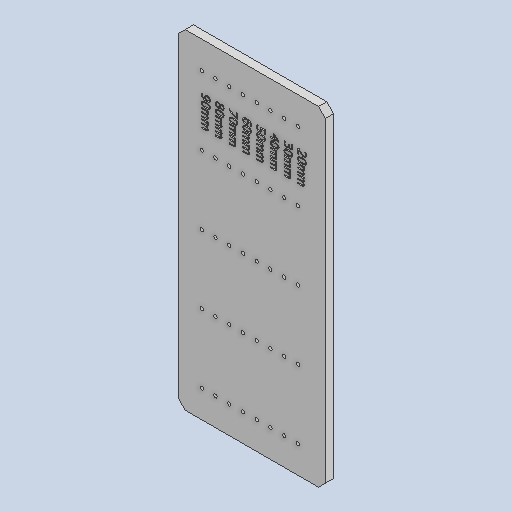
# Autodesk Inventor part: A-01
Saved by Autodesk Inventor 2022 (Build 260153000, 153)
## iProperties
Created: 2021-10-10
Part Number: A-01
Material: Generic
Document SubType Name: Modeling
Designer: kfcs7
Density: 1 g/cm^3
Appearance: Default
Author: kfcs7
Autodesk Inventor part; units mm, degrees
(part 1 of 2)
ref_plane "YZ Plane" through (0, 0, 0) normal (1, 0, 0) x (0, 1, 0)
ref_plane "XZ Plane" through (0, 0, 0) normal (0, 1, 0) x (-1, 0, 0)
ref_plane "XY Plane" through (0, 0, 0) normal (0, 0, 1) x (1, 0, 0)
sketch "Sketch1" plane through (0, 0, 0) normal (0, 0, 1) x (1, 0, 0)
  line L0 (14.5, -5) -> (14.5, -245) construction
  line L1 (14.5, -5) -> (0, -5) construction
  line L2 (0, -5) -> (0, -245) construction
  line L3 (0, -245) -> (14.5, -245) construction
  circle A0 centre (7, -25) radius 3.75 construction
  circle A1 centre (7, -75) radius 3.75 construction
  circle A2 centre (7, -125) radius 3.75 construction
  circle A3 centre (7, -175) radius 3.75 construction
  circle A4 centre (7, -225) radius 3.75 construction
  line L4 (27, -5) -> (-80, -5)
  line L5 (-80, -5) -> (-80, -245)
  line L6 (-80, -245) -> (27, -245)
  line L7 (27, -245) -> (27, -5)
  point P0 (0, 0)
  dimension "d6" = 20
  dimension "d9" = 80
  constraints: 8 end point, 2 collinear, 2 parallel, 1 horizontal, 1 perpendicular
  measures "d6" distance from line of L7 A0.centre
  measures "d9" distance between parallel lines of L2 L5
extrude "Extrusion1" add sketch "Sketch1" along normal blind 6
sketch "Sketch3" plane through (0, 0, 6) normal (0, 0, 1) x (1, 0, 0)
  line L0 (14.5, -5) -> (14.5, -245) construction
  line L1 (14.5, -5) -> (0, -5) construction
  line L2 (0, -5) -> (0, -245) construction
  line L3 (0, -245) -> (14.5, -245) construction
  circle A0 centre (7, -25) radius 3.75 construction
  circle A1 centre (7, -75) radius 3.75 construction
  circle A2 centre (7, -125) radius 3.75 construction
  circle A3 centre (7, -175) radius 3.75 construction
  circle A4 centre (7, -225) radius 3.75 construction
  circle A5 centre (7, -25) radius 1.25
  circle A6 centre (7, -75) radius 1.25
  circle A7 centre (7, -125) radius 1.25
  circle A8 centre (7, -175) radius 1.25
  circle A9 centre (7, -225) radius 1.25
  point P0 (0, 0)
  dimension "d10" = 2.5
  dimension "d11" = 2.5
  dimension "d12" = 2.5
  dimension "d13" = 2.5
  dimension "d14" = 2.5
  constraints: 5 centre point, 5 coincident
  measures "d10" diameter of A5
  measures "d11" diameter of A6
  measures "d12" diameter of A7
  measures "d13" diameter of A8
  measures "d14" diameter of A9
extrude "Extrusion2" cut sketch "Sketch3" against normal through all
chamfer "Chamfer1" distance 5 angle 45 4 edges at (27, -5, 3) (-80, -5, 3) (-80, -245, 3) (27, -245, 3)
pattern_linear "Rectangular Pattern1" count 8 spacing 10 along (-1, 0, 0) of "Extrusion2"
sketch "Sketch4" plane through (0, 0, 6) normal (0, 0, 1) x (1, 0, 0)
  circle A0 centre (7, -75) radius 1.25 construction
  circle A1 centre (7, -175) radius 1.25 construction
  circle A2 centre (7, -125) radius 1.25 construction
  circle A3 centre (7, -25) radius 1.25 construction
  circle A4 centre (7, -225) radius 1.25 construction
  line L0 (-80, -10) -> (-80, -240) construction
  line L1 (-75, -245) -> (22, -245) construction
  line L2 (27, -240) -> (27, -10) construction
  line L3 (22, -5) -> (-75, -5) construction
  circle A5 centre (7, -25) radius 1.25 construction
  circle A6 centre (7, -75) radius 1.25 construction
  line L4 (7, -25) -> (7, -75) construction
  line L5 (27, -240) -> (22, -245) construction
  line L6 (22, -5) -> (27, -10) construction
  line L7 (-80, -10) -> (-75, -5) construction
  line L8 (-75, -245) -> (-80, -240) construction
  circle A7 centre (-63, -75) radius 1.25 construction
  circle A8 centre (-63, -225) radius 1.25 construction
  circle A9 centre (-63, -25) radius 1.25 construction
  circle A10 centre (-63, -125) radius 1.25 construction
  circle A11 centre (-63, -175) radius 1.25 construction
  circle A12 centre (-53, -75) radius 1.25 construction
  circle A13 centre (-53, -225) radius 1.25 construction
  circle A14 centre (-53, -25) radius 1.25 construction
  circle A15 centre (-53, -125) radius 1.25 construction
  circle A16 centre (-53, -175) radius 1.25 construction
  circle A17 centre (-43, -75) radius 1.25 construction
  circle A18 centre (-43, -225) radius 1.25 construction
  circle A19 centre (-43, -25) radius 1.25 construction
  circle A20 centre (-43, -125) radius 1.25 construction
  circle A21 centre (-43, -175) radius 1.25 construction
  circle A22 centre (-33, -75) radius 1.25 construction
  circle A23 centre (-33, -225) radius 1.25 construction
  circle A24 centre (-33, -25) radius 1.25 construction
  circle A25 centre (-33, -125) radius 1.25 construction
  circle A26 centre (-33, -175) radius 1.25 construction
  circle A27 centre (-23, -75) radius 1.25 construction
  circle A28 centre (-23, -225) radius 1.25 construction
  circle A29 centre (-23, -25) radius 1.25 construction
  circle A30 centre (-23, -125) radius 1.25 construction
  circle A31 centre (-23, -175) radius 1.25 construction
  circle A32 centre (-13, -75) radius 1.25 construction
  circle A33 centre (-13, -225) radius 1.25 construction
  circle A34 centre (-13, -25) radius 1.25 construction
  circle A35 centre (-13, -125) radius 1.25 construction
  circle A36 centre (-13, -175) radius 1.25 construction
  circle A37 centre (-3, -75) radius 1.25 construction
  circle A38 centre (-3, -225) radius 1.25 construction
  circle A39 centre (-3, -25) radius 1.25 construction
  circle A40 centre (-3, -125) radius 1.25 construction
  circle A41 centre (-3, -175) radius 1.25 construction
  line L9 (27, -240) -> (22, -245) construction
  line L10 (27, -240) -> (27, -10) construction
  line L11 (22, -5) -> (27, -10) construction
  line L12 (22, -5) -> (-75, -5) construction
  line L13 (-80, -10) -> (-75, -5) construction
  line L14 (-80, -10) -> (-80, -240) construction
  line L15 (-75, -245) -> (-80, -240) construction
  line L16 (-75, -245) -> (22, -245) construction
  circle A42 centre (7, -75) radius 1.25 construction
  circle A43 centre (7, -175) radius 1.25 construction
  circle A44 centre (7, -125) radius 1.25 construction
  circle A45 centre (7, -25) radius 1.25 construction
  circle A46 centre (7, -225) radius 1.25 construction
  circle A47 centre (-3, -25) radius 1.25 construction
  line L17 (-3, -25) -> (-3, -75) construction
  circle A48 centre (-13, -75) radius 1.25 construction
  line L18 (-13, -25) -> (-13, -75) construction
  circle A49 centre (-23, -75) radius 1.25 construction
  circle A50 centre (-23, -25) radius 1.25 construction
  line L19 (-23, -75) -> (-23, -25) construction
  circle A51 centre (-33, -25) radius 1.25 construction
  circle A52 centre (-33, -75) radius 1.25 construction
  line L20 (-33, -25) -> (-33, -75) construction
  circle A53 centre (-43, -75) radius 1.25 construction
  circle A54 centre (-43, -25) radius 1.25 construction
  line L21 (-43, -75) -> (-43, -25) construction
  circle A55 centre (-53, -25) radius 1.25 construction
  circle A56 centre (-53, -75) radius 1.25 construction
  line L22 (-53, -25) -> (-53, -75) construction
  circle A57 centre (-63, -25) radius 1.25 construction
  circle A58 centre (-63, -75) radius 1.25 construction
  line L23 (-63, -25) -> (-63, -75) construction
  line L24 (7, -42.5851) -> (7, -38.8233)
  line L25 (7, -38.8233) -> (7.8651, -38.8233)
  spline S0 degree 2 poles (7.8651, -38.8233) (8.2457, -39.2286) (8.9526, -39.9503) (9.3332, -40.2964) knots 0 0 0 1 2 2 2
  spline S1 degree 2 poles (9.3332, -40.2964) (10.0994, -40.9934) (11.0189, -41.5025) (11.5083, -41.5025) knots 0 0 0 1 2 2 2
  spline S2 degree 2 poles (11.5083, -41.5025) (11.7653, -41.5025) (12.1509, -41.3443) (12.2745, -41.201) knots 0 0 0 1 2 2 2
  spline S3 degree 2 poles (12.2745, -41.201) (12.3981, -41.0576) (12.5216, -40.6819) (12.5216, -40.4545) knots 0 0 0 1 2 2 2
  spline S4 degree 2 poles (12.5216, -40.4545) (12.5216, -40.237) (12.4129, -39.7921) (12.3288, -39.5895) knots 0 0 0 1 2 2 2
  spline S5 degree 2 poles (12.3288, -39.5895) (12.2596, -39.4165) (12.0619, -39.0951) (11.9927, -38.9963) knots 0 0 0 1 2 2 2
  line L26 (11.9927, -38.9963) -> (11.9927, -38.9518)
  line L27 (11.9927, -38.9518) -> (12.8627, -38.9518)
  spline S6 degree 2 poles (12.8627, -38.9518) (12.9863, -39.2039) (13.2285, -40.1085) (13.2285, -40.5139) knots 0 0 0 1 2 2 2
  spline S7 degree 2 poles (13.2285, -40.5139) (13.2285, -41.369) (12.3239, -42.333) (11.5528, -42.333) knots 0 0 0 1 2 2 2
  spline S8 degree 2 poles (11.5528, -42.333) (11.1919, -42.333) (10.5888, -42.1649) (10.3318, -42.0166) knots 0 0 0 1 2 2 2
  spline S9 degree 2 poles (10.3318, -42.0166) (10.0648, -41.8683) (9.5408, -41.4382) (9.2887, -41.201) knots 0 0 0 1 2 2 2
  spline S10 degree 2 poles (9.2887, -41.201) (8.8686, -40.8154) (7.9689, -39.8712) (7.7069, -39.5895) knots 0 0 0 1 2 2 2
  line L28 (7.7069, -39.5895) -> (7.7069, -42.5851)
  line L29 (7.7069, -42.5851) -> (7, -42.5851)
  spline S11 degree 2 poles (10.05, -47.1972) (8.4088, -47.1972) (6.8715, -46.2431) (6.8715, -45.2495) knots 0 0 0 1 2 2 2
  spline S12 degree 2 poles (6.8715, -45.2495) (6.8715, -44.2411) (8.4385, -43.2969) (10.0451, -43.2969) knots 0 0 0 1 2 2 2
  spline S13 degree 2 poles (10.0451, -43.2969) (11.6961, -43.2969) (13.2236, -44.251) (13.2236, -45.2495) knots 0 0 0 1 2 2 2
  spline S14 degree 2 poles (13.2236, -45.2495) (13.2236, -46.253) (11.6417, -47.1972) (10.05, -47.1972) knots 0 0 0 1 2 2 2
  spline S15 degree 2 poles (8.1913, -46.1492) (8.4929, -46.2678) (9.4222, -46.3667) (10.05, -46.3667) knots 0 0 0 1 2 2 2
  spline S16 degree 2 poles (10.05, -46.3667) (10.6778, -46.3667) (11.6022, -46.2678) (11.9136, -46.1442) knots 0 0 0 1 2 2 2
  spline S17 degree 2 poles (11.9136, -46.1442) (12.225, -46.0207) (12.5464, -45.5906) (12.5464, -45.2495) knots 0 0 0 1 2 2 2
  spline S18 degree 2 poles (12.5464, -45.2495) (12.5464, -44.9084) (12.225, -44.4685) (11.9037, -44.34) knots 0 0 0 1 2 2 2
  spline S19 degree 2 poles (11.9037, -44.34) (11.5923, -44.2164) (10.6432, -44.1274) (10.0451, -44.1274) knots 0 0 0 1 2 2 2
  spline S20 degree 2 poles (10.0451, -44.1274) (9.4024, -44.1274) (8.5423, -44.2065) (8.2062, -44.335) knots 0 0 0 1 2 2 2
  spline S21 degree 2 poles (8.2062, -44.335) (7.8898, -44.4536) (7.5487, -44.8936) (7.5487, -45.2495) knots 0 0 0 1 2 2 2
  spline S22 degree 2 poles (7.5487, -45.2495) (7.5487, -45.5857) (7.87, -46.0256) (8.1913, -46.1492) knots 0 0 0 1 2 2 2
  line L30 (7, -53.2823) -> (9.6496, -53.2823)
  spline S23 degree 2 poles (9.6496, -53.2823) (9.966, -53.2823) (10.5048, -53.2329) (10.6531, -53.1538) knots 0 0 0 1 2 2 2
  spline S24 degree 2 poles (10.6531, -53.1538) (10.8162, -53.0747) (10.9744, -52.7732) (10.9744, -52.5112) knots 0 0 0 1 2 2 2
  spline S25 degree 2 poles (10.9744, -52.5112) (10.9744, -52.2739) (10.6827, -51.7301) (10.4059, -51.4434) knots 0 0 0 1 2 2 2
  spline S26 degree 2 poles (10.4059, -51.4434) (10.3367, -51.4484) (10.1439, -51.4583) (10.0154, -51.4583) knots 0 0 0 1 2 2 2
  line L31 (10.0154, -51.4583) -> (7, -51.4583)
  line L32 (7, -51.4583) -> (7, -50.6871)
  line L33 (7, -50.6871) -> (9.6496, -50.6871)
  spline S27 degree 2 poles (9.6496, -50.6871) (9.966, -50.6871) (10.5048, -50.6377) (10.6531, -50.5586) knots 0 0 0 1 2 2 2
  spline S28 degree 2 poles (10.6531, -50.5586) (10.8162, -50.4795) (10.9744, -50.178) (10.9744, -49.916) knots 0 0 0 1 2 2 2
  spline S29 degree 2 poles (10.9744, -49.916) (10.9744, -49.6688) (10.663, -49.1201) (10.4207, -48.863) knots 0 0 0 1 2 2 2
  line L34 (10.4207, -48.863) -> (7, -48.863)
  line L35 (7, -48.863) -> (7, -48.0919)
  line L36 (7, -48.0919) -> (11.5775, -48.0919)
  line L37 (11.5775, -48.0919) -> (11.5775, -48.863)
  line L38 (11.5775, -48.863) -> (11.0733, -48.863)
  spline S30 degree 2 poles (11.0733, -48.863) (11.3748, -49.1646) (11.706, -49.7578) (11.706, -50.1137) knots 0 0 0 1 2 2 2
  spline S31 degree 2 poles (11.706, -50.1137) (11.706, -50.519) (11.3353, -51.1468) (10.9151, -51.31) knots 0 0 0 1 2 2 2
  spline S32 degree 2 poles (10.9151, -51.31) (11.3056, -51.6609) (11.706, -52.3233) (11.706, -52.7089) knots 0 0 0 1 2 2 2
  spline S33 degree 2 poles (11.706, -52.7089) (11.706, -53.0055) (11.5231, -53.49) (11.3155, -53.6679) knots 0 0 0 1 2 2 2
  spline S34 degree 2 poles (11.3155, -53.6679) (11.1079, -53.8508) (10.485, -54.0535) (10.0154, -54.0535) knots 0 0 0 1 2 2 2
  line L39 (10.0154, -54.0535) -> (7, -54.0535)
  line L40 (7, -54.0535) -> (7, -53.2823)
  line L41 (7, -60.3265) -> (9.6496, -60.3265)
  spline S35 degree 2 poles (9.6496, -60.3265) (9.966, -60.3265) (10.5048, -60.2771) (10.6531, -60.198) knots 0 0 0 1 2 2 2
  spline S36 degree 2 poles (10.6531, -60.198) (10.8162, -60.1189) (10.9744, -59.8173) (10.9744, -59.5553) knots 0 0 0 1 2 2 2
  spline S37 degree 2 poles (10.9744, -59.5553) (10.9744, -59.3181) (10.6827, -58.7743) (10.4059, -58.4876) knots 0 0 0 1 2 2 2
  spline S38 degree 2 poles (10.4059, -58.4876) (10.3367, -58.4925) (10.1439, -58.5024) (10.0154, -58.5024) knots 0 0 0 1 2 2 2
  line L42 (10.0154, -58.5024) -> (7, -58.5024)
  line L43 (7, -58.5024) -> (7, -57.7313)
  line L44 (7, -57.7313) -> (9.6496, -57.7313)
  spline S39 degree 2 poles (9.6496, -57.7313) (9.966, -57.7313) (10.5048, -57.6818) (10.6531, -57.6028) knots 0 0 0 1 2 2 2
  spline S40 degree 2 poles (10.6531, -57.6028) (10.8162, -57.5237) (10.9744, -57.2221) (10.9744, -56.9601) knots 0 0 0 1 2 2 2
  spline S41 degree 2 poles (10.9744, -56.9601) (10.9744, -56.713) (10.663, -56.1643) (10.4207, -55.9072) knots 0 0 0 1 2 2 2
  line L45 (10.4207, -55.9072) -> (7, -55.9072)
  line L46 (7, -55.9072) -> (7, -55.1361)
  line L47 (7, -55.1361) -> (11.5775, -55.1361)
  line L48 (11.5775, -55.1361) -> (11.5775, -55.9072)
  line L49 (11.5775, -55.9072) -> (11.0733, -55.9072)
  spline S42 degree 2 poles (11.0733, -55.9072) (11.3748, -56.2088) (11.706, -56.8019) (11.706, -57.1579) knots 0 0 0 1 2 2 2
  spline S43 degree 2 poles (11.706, -57.1579) (11.706, -57.5632) (11.3353, -58.191) (10.9151, -58.3541) knots 0 0 0 1 2 2 2
  spline S44 degree 2 poles (10.9151, -58.3541) (11.3056, -58.7051) (11.706, -59.3675) (11.706, -59.7531) knots 0 0 0 1 2 2 2
  spline S45 degree 2 poles (11.706, -59.7531) (11.706, -60.0497) (11.5231, -60.5341) (11.3155, -60.7121) knots 0 0 0 1 2 2 2
  spline S46 degree 2 poles (11.3155, -60.7121) (11.1079, -60.895) (10.485, -61.0976) (10.0154, -61.0976) knots 0 0 0 1 2 2 2
  line L50 (10.0154, -61.0976) -> (7, -61.0976)
  line L51 (7, -61.0976) -> (7, -60.3265)
  spline S47 degree 2 poles (2.5216, -40.4694) (2.5216, -40.2469) (2.4129, -39.807) (2.3288, -39.5944) knots 0 0 0 1 2 2 2
  spline S48 degree 2 poles (2.3288, -39.5944) (2.2448, -39.3967) (2.0669, -39.105) (1.9878, -38.9913) knots 0 0 0 1 2 2 2
  line L52 (1.9878, -38.9913) -> (1.9878, -38.9419)
  line L53 (1.9878, -38.9419) -> (2.8528, -38.9419)
  spline S49 degree 2 poles (2.8528, -38.9419) (2.9962, -39.2088) (3.2285, -40.1233) (3.2285, -40.5336) knots 0 0 0 1 2 2 2
  spline S50 degree 2 poles (3.2285, -40.5336) (3.2285, -40.9489) (3.0605, -41.5668) (2.8825, -41.8189) knots 0 0 0 1 2 2 2
  spline S51 degree 2 poles (2.8825, -41.8189) (2.6897, -42.0858) (2.1311, -42.3626) (1.7554, -42.3626) knots 0 0 0 1 2 2 2
  spline S52 degree 2 poles (1.7554, -42.3626) (1.2512, -42.3626) (0.49, -41.7002) (0.3911, -41.2356) knots 0 0 0 1 2 2 2
  line L54 (0.3911, -41.2356) -> (0.3318, -41.2356)
  spline S53 degree 2 poles (0.3318, -41.2356) (0.2922, -41.4284) (0.1143, -41.8683) (-0.0637, -42.0562) knots 0 0 0 1 2 2 2
  spline S54 degree 2 poles (-0.0637, -42.0562) (-0.2367, -42.244) (-0.7904, -42.4813) (-1.1908, -42.4813) knots 0 0 0 1 2 2 2
  spline S55 degree 2 poles (-1.1908, -42.4813) (-1.6011, -42.4813) (-2.2981, -42.1995) (-2.565, -41.9425) knots 0 0 0 1 2 2 2
  spline S56 degree 2 poles (-2.565, -41.9425) (-2.8418, -41.6755) (-3.1285, -40.9192) (-3.1285, -40.4397) knots 0 0 0 1 2 2 2
  spline S57 degree 2 poles (-3.1285, -40.4397) (-3.1285, -39.98) (-2.9061, -39.0803) (-2.7528, -38.7738) knots 0 0 0 1 2 2 2
  line L55 (-2.7528, -38.7738) -> (-1.8878, -38.7738)
  line L56 (-1.8878, -38.7738) -> (-1.8878, -38.8331)
  spline S58 degree 2 poles (-1.8878, -38.8331) (-2.0756, -39.0902) (-2.4216, -39.9602) (-2.4216, -40.3903) knots 0 0 0 1 2 2 2
  spline S59 degree 2 poles (-2.4216, -40.3903) (-2.4216, -40.6424) (-2.2635, -41.1466) (-2.0806, -41.3147) knots 0 0 0 1 2 2 2
  spline S60 degree 2 poles (-2.0806, -41.3147) (-1.8976, -41.4778) (-1.4626, -41.6508) (-1.1314, -41.6508) knots 0 0 0 1 2 2 2
  spline S61 degree 2 poles (-1.1314, -41.6508) (-0.8002, -41.6508) (-0.3702, -41.458) (-0.2466, -41.285) knots 0 0 0 1 2 2 2
  spline S62 degree 2 poles (-0.2466, -41.285) (-0.123, -41.112) (-0.0291, -40.6424) (-0.0291, -40.3656) knots 0 0 0 1 2 2 2
  line L57 (-0.0291, -40.3656) -> (-0.0291, -40.0195)
  line L58 (-0.0291, -40.0195) -> (0.6481, -40.0195)
  line L59 (0.6481, -40.0195) -> (0.6481, -40.2914)
  spline S63 degree 2 poles (0.6481, -40.2914) (0.6481, -40.8401) (1.1721, -41.5322) (1.6714, -41.5322) knots 0 0 0 1 2 2 2
  spline S64 degree 2 poles (1.6714, -41.5322) (1.9037, -41.5322) (2.2349, -41.3542) (2.3338, -41.2109) knots 0 0 0 1 2 2 2
  spline S65 degree 2 poles (2.3338, -41.2109) (2.4376, -41.0576) (2.5216, -40.6819) (2.5216, -40.4694) knots 0 0 0 1 2 2 2
  spline S66 degree 2 poles (0.05, -47.1972) (-1.5912, -47.1972) (-3.1285, -46.2431) (-3.1285, -45.2495) knots 0 0 0 1 2 2 2
  spline S67 degree 2 poles (-3.1285, -45.2495) (-3.1285, -44.2411) (-1.5615, -43.2969) (0.0451, -43.2969) knots 0 0 0 1 2 2 2
  spline S68 degree 2 poles (0.0451, -43.2969) (1.6961, -43.2969) (3.2236, -44.251) (3.2236, -45.2495) knots 0 0 0 1 2 2 2
  spline S69 degree 2 poles (3.2236, -45.2495) (3.2236, -46.253) (1.6417, -47.1972) (0.05, -47.1972) knots 0 0 0 1 2 2 2
  spline S70 degree 2 poles (-1.8087, -46.1492) (-1.5071, -46.2678) (-0.5778, -46.3667) (0.05, -46.3667) knots 0 0 0 1 2 2 2
  spline S71 degree 2 poles (0.05, -46.3667) (0.6778, -46.3667) (1.6022, -46.2678) (1.9136, -46.1442) knots 0 0 0 1 2 2 2
  spline S72 degree 2 poles (1.9136, -46.1442) (2.225, -46.0207) (2.5464, -45.5906) (2.5464, -45.2495) knots 0 0 0 1 2 2 2
  spline S73 degree 2 poles (2.5464, -45.2495) (2.5464, -44.9084) (2.225, -44.4685) (1.9037, -44.34) knots 0 0 0 1 2 2 2
  spline S74 degree 2 poles (1.9037, -44.34) (1.5923, -44.2164) (0.6432, -44.1274) (0.0451, -44.1274) knots 0 0 0 1 2 2 2
  spline S75 degree 2 poles (0.0451, -44.1274) (-0.5976, -44.1274) (-1.4577, -44.2065) (-1.7938, -44.335) knots 0 0 0 1 2 2 2
  spline S76 degree 2 poles (-1.7938, -44.335) (-2.1102, -44.4536) (-2.4513, -44.8936) (-2.4513, -45.2495) knots 0 0 0 1 2 2 2
  spline S77 degree 2 poles (-2.4513, -45.2495) (-2.4513, -45.5857) (-2.13, -46.0256) (-1.8087, -46.1492) knots 0 0 0 1 2 2 2
  line L60 (-3, -53.2823) -> (-0.3504, -53.2823)
  spline S78 degree 2 poles (-0.3504, -53.2823) (-0.034, -53.2823) (0.5048, -53.2329) (0.6531, -53.1538) knots 0 0 0 1 2 2 2
  spline S79 degree 2 poles (0.6531, -53.1538) (0.8162, -53.0747) (0.9744, -52.7732) (0.9744, -52.5112) knots 0 0 0 1 2 2 2
  spline S80 degree 2 poles (0.9744, -52.5112) (0.9744, -52.2739) (0.6827, -51.7301) (0.4059, -51.4434) knots 0 0 0 1 2 2 2
  spline S81 degree 2 poles (0.4059, -51.4434) (0.3367, -51.4484) (0.1439, -51.4583) (0.0154, -51.4583) knots 0 0 0 1 2 2 2
  line L61 (0.0154, -51.4583) -> (-3, -51.4583)
  line L62 (-3, -51.4583) -> (-3, -50.6871)
  line L63 (-3, -50.6871) -> (-0.3504, -50.6871)
  spline S82 degree 2 poles (-0.3504, -50.6871) (-0.034, -50.6871) (0.5048, -50.6377) (0.6531, -50.5586) knots 0 0 0 1 2 2 2
  spline S83 degree 2 poles (0.6531, -50.5586) (0.8162, -50.4795) (0.9744, -50.178) (0.9744, -49.916) knots 0 0 0 1 2 2 2
  spline S84 degree 2 poles (0.9744, -49.916) (0.9744, -49.6688) (0.663, -49.1201) (0.4207, -48.863) knots 0 0 0 1 2 2 2
  line L64 (0.4207, -48.863) -> (-3, -48.863)
  line L65 (-3, -48.863) -> (-3, -48.0919)
  line L66 (-3, -48.0919) -> (1.5775, -48.0919)
  line L67 (1.5775, -48.0919) -> (1.5775, -48.863)
  line L68 (1.5775, -48.863) -> (1.0733, -48.863)
  spline S85 degree 2 poles (1.0733, -48.863) (1.3748, -49.1646) (1.706, -49.7578) (1.706, -50.1137) knots 0 0 0 1 2 2 2
  spline S86 degree 2 poles (1.706, -50.1137) (1.706, -50.519) (1.3353, -51.1468) (0.9151, -51.31) knots 0 0 0 1 2 2 2
  spline S87 degree 2 poles (0.9151, -51.31) (1.3056, -51.6609) (1.706, -52.3233) (1.706, -52.7089) knots 0 0 0 1 2 2 2
  spline S88 degree 2 poles (1.706, -52.7089) (1.706, -53.0055) (1.5231, -53.49) (1.3155, -53.6679) knots 0 0 0 1 2 2 2
  spline S89 degree 2 poles (1.3155, -53.6679) (1.1079, -53.8508) (0.485, -54.0535) (0.0154, -54.0535) knots 0 0 0 1 2 2 2
  line L69 (0.0154, -54.0535) -> (-3, -54.0535)
  line L70 (-3, -54.0535) -> (-3, -53.2823)
  line L71 (-3, -60.3265) -> (-0.3504, -60.3265)
  spline S90 degree 2 poles (-0.3504, -60.3265) (-0.034, -60.3265) (0.5048, -60.2771) (0.6531, -60.198) knots 0 0 0 1 2 2 2
  spline S91 degree 2 poles (0.6531, -60.198) (0.8162, -60.1189) (0.9744, -59.8173) (0.9744, -59.5553) knots 0 0 0 1 2 2 2
  spline S92 degree 2 poles (0.9744, -59.5553) (0.9744, -59.3181) (0.6827, -58.7743) (0.4059, -58.4876) knots 0 0 0 1 2 2 2
  spline S93 degree 2 poles (0.4059, -58.4876) (0.3367, -58.4925) (0.1439, -58.5024) (0.0154, -58.5024) knots 0 0 0 1 2 2 2
  line L72 (0.0154, -58.5024) -> (-3, -58.5024)
  line L73 (-3, -58.5024) -> (-3, -57.7313)
  line L74 (-3, -57.7313) -> (-0.3504, -57.7313)
  spline S94 degree 2 poles (-0.3504, -57.7313) (-0.034, -57.7313) (0.5048, -57.6818) (0.6531, -57.6028) knots 0 0 0 1 2 2 2
  spline S95 degree 2 poles (0.6531, -57.6028) (0.8162, -57.5237) (0.9744, -57.2221) (0.9744, -56.9601) knots 0 0 0 1 2 2 2
  spline S96 degree 2 poles (0.9744, -56.9601) (0.9744, -56.713) (0.663, -56.1643) (0.4207, -55.9072) knots 0 0 0 1 2 2 2
  line L75 (0.4207, -55.9072) -> (-3, -55.9072)
  line L76 (-3, -55.9072) -> (-3, -55.1361)
  line L77 (-3, -55.1361) -> (1.5775, -55.1361)
  line L78 (1.5775, -55.1361) -> (1.5775, -55.9072)
  line L79 (1.5775, -55.9072) -> (1.0733, -55.9072)
  spline S97 degree 2 poles (1.0733, -55.9072) (1.3748, -56.2088) (1.706, -56.8019) (1.706, -57.1579) knots 0 0 0 1 2 2 2
  spline S98 degree 2 poles (1.706, -57.1579) (1.706, -57.5632) (1.3353, -58.191) (0.9151, -58.3541) knots 0 0 0 1 2 2 2
  spline S99 degree 2 poles (0.9151, -58.3541) (1.3056, -58.7051) (1.706, -59.3675) (1.706, -59.7531) knots 0 0 0 1 2 2 2
  spline S100 degree 2 poles (1.706, -59.7531) (1.706, -60.0497) (1.5231, -60.5341) (1.3155, -60.7121) knots 0 0 0 1 2 2 2
  spline S101 degree 2 poles (1.3155, -60.7121) (1.1079, -60.895) (0.485, -61.0976) (0.0154, -61.0976) knots 0 0 0 1 2 2 2
  line L80 (0.0154, -61.0976) -> (-3, -61.0976)
  line L81 (-3, -61.0976) -> (-3, -60.3265)
  line L82 (-10.9041, -42.7482) -> (-10.9041, -42.0216)
  line L83 (-10.9041, -42.0216) -> (-13, -42.0216)
  line L84 (-13, -42.0216) -> (-13, -41.2356)
  line L85 (-13, -41.2356) -> (-10.9041, -41.2356)
  line L86 (-10.9041, -41.2356) -> (-10.9041, -38.5415)
  line L87 (-10.9041, -38.5415) -> (-10.0439, -38.5415)
  line L88 (-10.0439, -38.5415) -> (-6.9, -41.2702)
  line L89 (-6.9, -41.2702) -> (-6.9, -42.0216)
  line L90 (-6.9, -42.0216) -> (-10.2466, -42.0216)
  line L91 (-10.2466, -42.0216) -> (-10.2466, -42.7482)
  line L92 (-10.2466, -42.7482) -> (-10.9041, -42.7482)
  line L93 (-10.2466, -41.2356) -> (-7.8639, -41.2356)
  line L94 (-7.8639, -41.2356) -> (-10.2466, -39.1841)
  line L95 (-10.2466, -39.1841) -> (-10.2466, -41.2356)
  spline S102 degree 2 poles (-9.95, -47.1972) (-11.5912, -47.1972) (-13.1285, -46.2431) (-13.1285, -45.2495) knots 0 0 0 1 2 2 2
  spline S103 degree 2 poles (-13.1285, -45.2495) (-13.1285, -44.2411) (-11.5615, -43.2969) (-9.9549, -43.2969) knots 0 0 0 1 2 2 2
  spline S104 degree 2 poles (-9.9549, -43.2969) (-8.3039, -43.2969) (-6.7764, -44.251) (-6.7764, -45.2495) knots 0 0 0 1 2 2 2
  spline S105 degree 2 poles (-6.7764, -45.2495) (-6.7764, -46.253) (-8.3583, -47.1972) (-9.95, -47.1972) knots 0 0 0 1 2 2 2
  spline S106 degree 2 poles (-11.8087, -46.1492) (-11.5071, -46.2678) (-10.5778, -46.3667) (-9.95, -46.3667) knots 0 0 0 1 2 2 2
  spline S107 degree 2 poles (-9.95, -46.3667) (-9.3222, -46.3667) (-8.3978, -46.2678) (-8.0864, -46.1442) knots 0 0 0 1 2 2 2
  spline S108 degree 2 poles (-8.0864, -46.1442) (-7.775, -46.0207) (-7.4536, -45.5906) (-7.4536, -45.2495) knots 0 0 0 1 2 2 2
  spline S109 degree 2 poles (-7.4536, -45.2495) (-7.4536, -44.9084) (-7.775, -44.4685) (-8.0963, -44.34) knots 0 0 0 1 2 2 2
  spline S110 degree 2 poles (-8.0963, -44.34) (-8.4077, -44.2164) (-9.3568, -44.1274) (-9.9549, -44.1274) knots 0 0 0 1 2 2 2
  spline S111 degree 2 poles (-9.9549, -44.1274) (-10.5976, -44.1274) (-11.4577, -44.2065) (-11.7938, -44.335) knots 0 0 0 1 2 2 2
  spline S112 degree 2 poles (-11.7938, -44.335) (-12.1102, -44.4536) (-12.4513, -44.8936) (-12.4513, -45.2495) knots 0 0 0 1 2 2 2
  spline S113 degree 2 poles (-12.4513, -45.2495) (-12.4513, -45.5857) (-12.13, -46.0256) (-11.8087, -46.1492) knots 0 0 0 1 2 2 2
  line L96 (-13, -53.2823) -> (-10.3504, -53.2823)
  spline S114 degree 2 poles (-10.3504, -53.2823) (-10.034, -53.2823) (-9.4952, -53.2329) (-9.3469, -53.1538) knots 0 0 0 1 2 2 2
  spline S115 degree 2 poles (-9.3469, -53.1538) (-9.1838, -53.0747) (-9.0256, -52.7732) (-9.0256, -52.5112) knots 0 0 0 1 2 2 2
  spline S116 degree 2 poles (-9.0256, -52.5112) (-9.0256, -52.2739) (-9.3173, -51.7301) (-9.5941, -51.4434) knots 0 0 0 1 2 2 2
  spline S117 degree 2 poles (-9.5941, -51.4434) (-9.6633, -51.4484) (-9.8561, -51.4583) (-9.9846, -51.4583) knots 0 0 0 1 2 2 2
  line L97 (-9.9846, -51.4583) -> (-13, -51.4583)
  line L98 (-13, -51.4583) -> (-13, -50.6871)
  line L99 (-13, -50.6871) -> (-10.3504, -50.6871)
  spline S118 degree 2 poles (-10.3504, -50.6871) (-10.034, -50.6871) (-9.4952, -50.6377) (-9.3469, -50.5586) knots 0 0 0 1 2 2 2
  spline S119 degree 2 poles (-9.3469, -50.5586) (-9.1838, -50.4795) (-9.0256, -50.178) (-9.0256, -49.916) knots 0 0 0 1 2 2 2
  spline S120 degree 2 poles (-9.0256, -49.916) (-9.0256, -49.6688) (-9.337, -49.1201) (-9.5793, -48.863) knots 0 0 0 1 2 2 2
  line L100 (-9.5793, -48.863) -> (-13, -48.863)
  line L101 (-13, -48.863) -> (-13, -48.0919)
  line L102 (-13, -48.0919) -> (-8.4225, -48.0919)
  line L103 (-8.4225, -48.0919) -> (-8.4225, -48.863)
  line L104 (-8.4225, -48.863) -> (-8.9267, -48.863)
  spline S121 degree 2 poles (-8.9267, -48.863) (-8.6252, -49.1646) (-8.294, -49.7578) (-8.294, -50.1137) knots 0 0 0 1 2 2 2
  spline S122 degree 2 poles (-8.294, -50.1137) (-8.294, -50.519) (-8.6647, -51.1468) (-9.0849, -51.31) knots 0 0 0 1 2 2 2
  spline S123 degree 2 poles (-9.0849, -51.31) (-8.6944, -51.6609) (-8.294, -52.3233) (-8.294, -52.7089) knots 0 0 0 1 2 2 2
  spline S124 degree 2 poles (-8.294, -52.7089) (-8.294, -53.0055) (-8.4769, -53.49) (-8.6845, -53.6679) knots 0 0 0 1 2 2 2
  spline S125 degree 2 poles (-8.6845, -53.6679) (-8.8921, -53.8508) (-9.515, -54.0535) (-9.9846, -54.0535) knots 0 0 0 1 2 2 2
  line L105 (-9.9846, -54.0535) -> (-13, -54.0535)
  line L106 (-13, -54.0535) -> (-13, -53.2823)
  line L107 (-13, -60.3265) -> (-10.3504, -60.3265)
  spline S126 degree 2 poles (-10.3504, -60.3265) (-10.034, -60.3265) (-9.4952, -60.2771) (-9.3469, -60.198) knots 0 0 0 1 2 2 2
  spline S127 degree 2 poles (-9.3469, -60.198) (-9.1838, -60.1189) (-9.0256, -59.8173) (-9.0256, -59.5553) knots 0 0 0 1 2 2 2
  spline S128 degree 2 poles (-9.0256, -59.5553) (-9.0256, -59.3181) (-9.3173, -58.7743) (-9.5941, -58.4876) knots 0 0 0 1 2 2 2
  spline S129 degree 2 poles (-9.5941, -58.4876) (-9.6633, -58.4925) (-9.8561, -58.5024) (-9.9846, -58.5024) knots 0 0 0 1 2 2 2
  line L108 (-9.9846, -58.5024) -> (-13, -58.5024)
  line L109 (-13, -58.5024) -> (-13, -57.7313)
  line L110 (-13, -57.7313) -> (-10.3504, -57.7313)
  spline S130 degree 2 poles (-10.3504, -57.7313) (-10.034, -57.7313) (-9.4952, -57.6818) (-9.3469, -57.6028) knots 0 0 0 1 2 2 2
  spline S131 degree 2 poles (-9.3469, -57.6028) (-9.1838, -57.5237) (-9.0256, -57.2221) (-9.0256, -56.9601) knots 0 0 0 1 2 2 2
  spline S132 degree 2 poles (-9.0256, -56.9601) (-9.0256, -56.713) (-9.337, -56.1643) (-9.5793, -55.9072) knots 0 0 0 1 2 2 2
  line L111 (-9.5793, -55.9072) -> (-13, -55.9072)
  line L112 (-13, -55.9072) -> (-13, -55.1361)
  line L113 (-13, -55.1361) -> (-8.4225, -55.1361)
  line L114 (-8.4225, -55.1361) -> (-8.4225, -55.9072)
  line L115 (-8.4225, -55.9072) -> (-8.9267, -55.9072)
  spline S133 degree 2 poles (-8.9267, -55.9072) (-8.6252, -56.2088) (-8.294, -56.8019) (-8.294, -57.1579) knots 0 0 0 1 2 2 2
  spline S134 degree 2 poles (-8.294, -57.1579) (-8.294, -57.5632) (-8.6647, -58.191) (-9.0849, -58.3541) knots 0 0 0 1 2 2 2
  spline S135 degree 2 poles (-9.0849, -58.3541) (-8.6944, -58.7051) (-8.294, -59.3675) (-8.294, -59.7531) knots 0 0 0 1 2 2 2
  spline S136 degree 2 poles (-8.294, -59.7531) (-8.294, -60.0497) (-8.4769, -60.5341) (-8.6845, -60.7121) knots 0 0 0 1 2 2 2
  spline S137 degree 2 poles (-8.6845, -60.7121) (-8.8921, -60.895) (-9.515, -61.0976) (-9.9846, -61.0976) knots 0 0 0 1 2 2 2
  line L116 (-9.9846, -61.0976) -> (-13, -61.0976)
  line L117 (-13, -61.0976) -> (-13, -60.3265)
  spline S138 degree 2 poles (-21.0622, -42.5208) (-21.5022, -42.5208) (-22.2536, -42.2391) (-22.5304, -41.982) knots 0 0 0 1 2 2 2
  spline S139 degree 2 poles (-22.5304, -41.982) (-22.8072, -41.725) (-23.1285, -40.9588) (-23.1285, -40.4842) knots 0 0 0 1 2 2 2
  spline S140 degree 2 poles (-23.1285, -40.4842) (-23.1285, -40.0492) (-22.9357, -39.1989) (-22.7825, -38.8875) knots 0 0 0 1 2 2 2
  line L118 (-22.7825, -38.8875) -> (-21.9174, -38.8875)
  line L119 (-21.9174, -38.8875) -> (-21.9174, -38.9468)
  spline S141 degree 2 poles (-21.9174, -38.9468) (-21.9866, -39.0408) (-22.1646, -39.3917) (-22.2437, -39.6043) knots 0 0 0 1 2 2 2
  spline S142 degree 2 poles (-22.2437, -39.6043) (-22.3277, -39.8465) (-22.4216, -40.2469) (-22.4216, -40.499) knots 0 0 0 1 2 2 2
  spline S143 degree 2 poles (-22.4216, -40.499) (-22.4216, -40.7462) (-22.2437, -41.2109) (-22.0509, -41.3789) knots 0 0 0 1 2 2 2
  spline S144 degree 2 poles (-22.0509, -41.3789) (-21.868, -41.5322) (-21.3835, -41.6904) (-21.0573, -41.6904) knots 0 0 0 1 2 2 2
  spline S145 degree 2 poles (-21.0573, -41.6904) (-20.731, -41.6904) (-20.3158, -41.5124) (-20.1774, -41.3443) knots 0 0 0 1 2 2 2
  spline S146 degree 2 poles (-20.1774, -41.3443) (-20.0241, -41.1713) (-19.8956, -40.6572) (-19.8956, -40.3458) knots 0 0 0 1 2 2 2
  spline S147 degree 2 poles (-19.8956, -40.3458) (-19.8956, -40.0096) (-19.9994, -39.3423) (-20.0439, -39.1396) knots 0 0 0 1 2 2 2
  line L120 (-20.0439, -39.1396) -> (-16.9, -39.1396)
  line L121 (-16.9, -39.1396) -> (-16.9, -42.4862)
  line L122 (-16.9, -42.4862) -> (-17.6168, -42.4862)
  line L123 (-17.6168, -42.4862) -> (-17.6168, -39.9256)
  line L124 (-17.6168, -39.9256) -> (-19.2431, -39.9256)
  spline S148 degree 2 poles (-19.2431, -39.9256) (-19.2233, -40.0739) (-19.2085, -40.3606) (-19.2085, -40.4793) knots 0 0 0 1 2 2 2
  spline S149 degree 2 poles (-19.2085, -40.4793) (-19.2085, -40.9489) (-19.3618, -41.5964) (-19.5891, -41.893) knots 0 0 0 1 2 2 2
  spline S150 degree 2 poles (-19.5891, -41.893) (-19.8165, -42.1946) (-20.5086, -42.5208) (-21.0622, -42.5208) knots 0 0 0 1 2 2 2
  spline S151 degree 2 poles (-19.95, -47.1972) (-21.5912, -47.1972) (-23.1285, -46.2431) (-23.1285, -45.2495) knots 0 0 0 1 2 2 2
  spline S152 degree 2 poles (-23.1285, -45.2495) (-23.1285, -44.2411) (-21.5615, -43.2969) (-19.9549, -43.2969) knots 0 0 0 1 2 2 2
  spline S153 degree 2 poles (-19.9549, -43.2969) (-18.3039, -43.2969) (-16.7764, -44.251) (-16.7764, -45.2495) knots 0 0 0 1 2 2 2
  spline S154 degree 2 poles (-16.7764, -45.2495) (-16.7764, -46.253) (-18.3583, -47.1972) (-19.95, -47.1972) knots 0 0 0 1 2 2 2
  spline S155 degree 2 poles (-21.8087, -46.1492) (-21.5071, -46.2678) (-20.5778, -46.3667) (-19.95, -46.3667) knots 0 0 0 1 2 2 2
  spline S156 degree 2 poles (-19.95, -46.3667) (-19.3222, -46.3667) (-18.3978, -46.2678) (-18.0864, -46.1442) knots 0 0 0 1 2 2 2
  spline S157 degree 2 poles (-18.0864, -46.1442) (-17.775, -46.0207) (-17.4536, -45.5906) (-17.4536, -45.2495) knots 0 0 0 1 2 2 2
  spline S158 degree 2 poles (-17.4536, -45.2495) (-17.4536, -44.9084) (-17.775, -44.4685) (-18.0963, -44.34) knots 0 0 0 1 2 2 2
  spline S159 degree 2 poles (-18.0963, -44.34) (-18.4077, -44.2164) (-19.3568, -44.1274) (-19.9549, -44.1274) knots 0 0 0 1 2 2 2
  spline S160 degree 2 poles (-19.9549, -44.1274) (-20.5976, -44.1274) (-21.4577, -44.2065) (-21.7938, -44.335) knots 0 0 0 1 2 2 2
  spline S161 degree 2 poles (-21.7938, -44.335) (-22.1102, -44.4536) (-22.4513, -44.8936) (-22.4513, -45.2495) knots 0 0 0 1 2 2 2
  spline S162 degree 2 poles (-22.4513, -45.2495) (-22.4513, -45.5857) (-22.13, -46.0256) (-21.8087, -46.1492) knots 0 0 0 1 2 2 2
  line L125 (-23, -53.2823) -> (-20.3504, -53.2823)
  spline S163 degree 2 poles (-20.3504, -53.2823) (-20.034, -53.2823) (-19.4952, -53.2329) (-19.3469, -53.1538) knots 0 0 0 1 2 2 2
  spline S164 degree 2 poles (-19.3469, -53.1538) (-19.1838, -53.0747) (-19.0256, -52.7732) (-19.0256, -52.5112) knots 0 0 0 1 2 2 2
  spline S165 degree 2 poles (-19.0256, -52.5112) (-19.0256, -52.2739) (-19.3173, -51.7301) (-19.5941, -51.4434) knots 0 0 0 1 2 2 2
  spline S166 degree 2 poles (-19.5941, -51.4434) (-19.6633, -51.4484) (-19.8561, -51.4583) (-19.9846, -51.4583) knots 0 0 0 1 2 2 2
  line L126 (-19.9846, -51.4583) -> (-23, -51.4583)
  line L127 (-23, -51.4583) -> (-23, -50.6871)
  line L128 (-23, -50.6871) -> (-20.3504, -50.6871)
  spline S167 degree 2 poles (-20.3504, -50.6871) (-20.034, -50.6871) (-19.4952, -50.6377) (-19.3469, -50.5586) knots 0 0 0 1 2 2 2
  spline S168 degree 2 poles (-19.3469, -50.5586) (-19.1838, -50.4795) (-19.0256, -50.178) (-19.0256, -49.916) knots 0 0 0 1 2 2 2
  spline S169 degree 2 poles (-19.0256, -49.916) (-19.0256, -49.6688) (-19.337, -49.1201) (-19.5793, -48.863) knots 0 0 0 1 2 2 2
  line L129 (-19.5793, -48.863) -> (-23, -48.863)
  line L130 (-23, -48.863) -> (-23, -48.0919)
  line L131 (-23, -48.0919) -> (-18.4225, -48.0919)
  line L132 (-18.4225, -48.0919) -> (-18.4225, -48.863)
  line L133 (-18.4225, -48.863) -> (-18.9267, -48.863)
  spline S170 degree 2 poles (-18.9267, -48.863) (-18.6252, -49.1646) (-18.294, -49.7578) (-18.294, -50.1137) knots 0 0 0 1 2 2 2
  spline S171 degree 2 poles (-18.294, -50.1137) (-18.294, -50.519) (-18.6647, -51.1468) (-19.0849, -51.31) knots 0 0 0 1 2 2 2
  spline S172 degree 2 poles (-19.0849, -51.31) (-18.6944, -51.6609) (-18.294, -52.3233) (-18.294, -52.7089) knots 0 0 0 1 2 2 2
  spline S173 degree 2 poles (-18.294, -52.7089) (-18.294, -53.0055) (-18.4769, -53.49) (-18.6845, -53.6679) knots 0 0 0 1 2 2 2
  spline S174 degree 2 poles (-18.6845, -53.6679) (-18.8921, -53.8508) (-19.515, -54.0535) (-19.9846, -54.0535) knots 0 0 0 1 2 2 2
  line L134 (-19.9846, -54.0535) -> (-23, -54.0535)
  line L135 (-23, -54.0535) -> (-23, -53.2823)
  line L136 (-23, -60.3265) -> (-20.3504, -60.3265)
  spline S175 degree 2 poles (-20.3504, -60.3265) (-20.034, -60.3265) (-19.4952, -60.2771) (-19.3469, -60.198) knots 0 0 0 1 2 2 2
  spline S176 degree 2 poles (-19.3469, -60.198) (-19.1838, -60.1189) (-19.0256, -59.8173) (-19.0256, -59.5553) knots 0 0 0 1 2 2 2
  spline S177 degree 2 poles (-19.0256, -59.5553) (-19.0256, -59.3181) (-19.3173, -58.7743) (-19.5941, -58.4876) knots 0 0 0 1 2 2 2
  spline S178 degree 2 poles (-19.5941, -58.4876) (-19.6633, -58.4925) (-19.8561, -58.5024) (-19.9846, -58.5024) knots 0 0 0 1 2 2 2
  line L137 (-19.9846, -58.5024) -> (-23, -58.5024)
  line L138 (-23, -58.5024) -> (-23, -57.7313)
  line L139 (-23, -57.7313) -> (-20.3504, -57.7313)
  spline S179 degree 2 poles (-20.3504, -57.7313) (-20.034, -57.7313) (-19.4952, -57.6818) (-19.3469, -57.6028) knots 0 0 0 1 2 2 2
  spline S180 degree 2 poles (-19.3469, -57.6028) (-19.1838, -57.5237) (-19.0256, -57.2221) (-19.0256, -56.9601) knots 0 0 0 1 2 2 2
  spline S181 degree 2 poles (-19.0256, -56.9601) (-19.0256, -56.713) (-19.337, -56.1643) (-19.5793, -55.9072) knots 0 0 0 1 2 2 2
  line L140 (-19.5793, -55.9072) -> (-23, -55.9072)
  line L141 (-23, -55.9072) -> (-23, -55.1361)
  line L142 (-23, -55.1361) -> (-18.4225, -55.1361)
  line L143 (-18.4225, -55.1361) -> (-18.4225, -55.9072)
  line L144 (-18.4225, -55.9072) -> (-18.9267, -55.9072)
  spline S182 degree 2 poles (-18.9267, -55.9072) (-18.6252, -56.2088) (-18.294, -56.8019) (-18.294, -57.1579) knots 0 0 0 1 2 2 2
  spline S183 degree 2 poles (-18.294, -57.1579) (-18.294, -57.5632) (-18.6647, -58.191) (-19.0849, -58.3541) knots 0 0 0 1 2 2 2
  spline S184 degree 2 poles (-19.0849, -58.3541) (-18.6944, -58.7051) (-18.294, -59.3675) (-18.294, -59.7531) knots 0 0 0 1 2 2 2
  spline S185 degree 2 poles (-18.294, -59.7531) (-18.294, -60.0497) (-18.4769, -60.5341) (-18.6845, -60.7121) knots 0 0 0 1 2 2 2
  spline S186 degree 2 poles (-18.6845, -60.7121) (-18.8921, -60.895) (-19.515, -61.0976) (-19.9846, -61.0976) knots 0 0 0 1 2 2 2
  line L145 (-19.9846, -61.0976) -> (-23, -61.0976)
  line L146 (-23, -61.0976) -> (-23, -60.3265)
  spline S187 degree 2 poles (-31.0227, -42.679) (-31.4923, -42.679) (-32.2882, -42.3676) (-32.5551, -42.1056) knots 0 0 0 1 2 2 2
  spline S188 degree 2 poles (-32.5551, -42.1056) (-32.8369, -41.8337) (-33.1285, -41.1515) (-33.1285, -40.7412) knots 0 0 0 1 2 2 2
  spline S189 degree 2 poles (-33.1285, -40.7412) (-33.1285, -40.331) (-32.8517, -39.6537) (-32.5749, -39.3967) knots 0 0 0 1 2 2 2
  spline S190 degree 2 poles (-32.5749, -39.3967) (-32.2437, -39.0803) (-31.1314, -38.7244) (-30.3207, -38.7244) knots 0 0 0 1 2 2 2
  spline S191 degree 2 poles (-30.3207, -38.7244) (-29.5249, -38.7244) (-28.2446, -39.0506) (-27.77, -39.3917) knots 0 0 0 1 2 2 2
  spline S192 degree 2 poles (-27.77, -39.3917) (-27.3053, -39.7229) (-26.7863, -40.7709) (-26.7863, -41.458) knots 0 0 0 1 2 2 2
  spline S193 degree 2 poles (-26.7863, -41.458) (-26.7863, -41.6607) (-26.8259, -42.0166) (-26.8703, -42.1501) knots 0 0 0 1 2 2 2
  line L147 (-26.8703, -42.1501) -> (-27.6563, -42.1501)
  line L148 (-27.6563, -42.1501) -> (-27.6563, -42.1155)
  spline S194 degree 2 poles (-27.6563, -42.1155) (-27.597, -42.0018) (-27.4932, -41.5865) (-27.4932, -41.3493) knots 0 0 0 1 2 2 2
  spline S195 degree 2 poles (-27.4932, -41.3493) (-27.4932, -40.588) (-28.5214, -39.6537) (-29.5298, -39.5647) knots 0 0 0 1 2 2 2
  spline S196 degree 2 poles (-29.5298, -39.5647) (-29.3271, -39.8564) (-29.1047, -40.4694) (-29.1047, -40.8352) knots 0 0 0 1 2 2 2
  spline S197 degree 2 poles (-29.1047, -40.8352) (-29.1047, -41.1911) (-29.2481, -41.725) (-29.4656, -42.0166) knots 0 0 0 1 2 2 2
  spline S198 degree 2 poles (-29.4656, -42.0166) (-29.7177, -42.3528) (-30.4987, -42.679) (-31.0227, -42.679) knots 0 0 0 1 2 2 2
  spline S199 degree 2 poles (-31.0573, -41.8485) (-30.6816, -41.8485) (-30.1724, -41.6508) (-29.9945, -41.4333) knots 0 0 0 1 2 2 2
  spline S200 degree 2 poles (-29.9945, -41.4333) (-29.866, -41.2702) (-29.7819, -40.8648) (-29.7819, -40.6523) knots 0 0 0 1 2 2 2
  spline S201 degree 2 poles (-29.7819, -40.6523) (-29.7819, -40.3656) (-29.9549, -39.8267) (-30.1181, -39.5647) knots 0 0 0 1 2 2 2
  spline S202 degree 2 poles (-30.1181, -39.5647) (-30.2071, -39.5598) (-30.3751, -39.5499) (-30.5036, -39.5499) knots 0 0 0 1 2 2 2
  spline S203 degree 2 poles (-30.5036, -39.5499) (-31.1364, -39.5499) (-31.9125, -39.7971) (-32.1152, -39.9849) knots 0 0 0 1 2 2 2
  spline S204 degree 2 poles (-32.1152, -39.9849) (-32.3079, -40.1579) (-32.4612, -40.5336) (-32.4612, -40.7462) knots 0 0 0 1 2 2 2
  spline S205 degree 2 poles (-32.4612, -40.7462) (-32.4612, -41.2405) (-31.7592, -41.8485) (-31.0573, -41.8485) knots 0 0 0 1 2 2 2
  spline S206 degree 2 poles (-29.95, -47.1972) (-31.5912, -47.1972) (-33.1285, -46.2431) (-33.1285, -45.2495) knots 0 0 0 1 2 2 2
  spline S207 degree 2 poles (-33.1285, -45.2495) (-33.1285, -44.2411) (-31.5615, -43.2969) (-29.9549, -43.2969) knots 0 0 0 1 2 2 2
  spline S208 degree 2 poles (-29.9549, -43.2969) (-28.3039, -43.2969) (-26.7764, -44.251) (-26.7764, -45.2495) knots 0 0 0 1 2 2 2
  spline S209 degree 2 poles (-26.7764, -45.2495) (-26.7764, -46.253) (-28.3583, -47.1972) (-29.95, -47.1972) knots 0 0 0 1 2 2 2
  spline S210 degree 2 poles (-31.8087, -46.1492) (-31.5071, -46.2678) (-30.5778, -46.3667) (-29.95, -46.3667) knots 0 0 0 1 2 2 2
  spline S211 degree 2 poles (-29.95, -46.3667) (-29.3222, -46.3667) (-28.3978, -46.2678) (-28.0864, -46.1442) knots 0 0 0 1 2 2 2
  spline S212 degree 2 poles (-28.0864, -46.1442) (-27.775, -46.0207) (-27.4536, -45.5906) (-27.4536, -45.2495) knots 0 0 0 1 2 2 2
  spline S213 degree 2 poles (-27.4536, -45.2495) (-27.4536, -44.9084) (-27.775, -44.4685) (-28.0963, -44.34) knots 0 0 0 1 2 2 2
  spline S214 degree 2 poles (-28.0963, -44.34) (-28.4077, -44.2164) (-29.3568, -44.1274) (-29.9549, -44.1274) knots 0 0 0 1 2 2 2
  spline S215 degree 2 poles (-29.9549, -44.1274) (-30.5976, -44.1274) (-31.4577, -44.2065) (-31.7938, -44.335) knots 0 0 0 1 2 2 2
  spline S216 degree 2 poles (-31.7938, -44.335) (-32.1102, -44.4536) (-32.4513, -44.8936) (-32.4513, -45.2495) knots 0 0 0 1 2 2 2
  spline S217 degree 2 poles (-32.4513, -45.2495) (-32.4513, -45.5857) (-32.13, -46.0256) (-31.8087, -46.1492) knots 0 0 0 1 2 2 2
  line L149 (-33, -53.2823) -> (-30.3504, -53.2823)
  spline S218 degree 2 poles (-30.3504, -53.2823) (-30.034, -53.2823) (-29.4952, -53.2329) (-29.3469, -53.1538) knots 0 0 0 1 2 2 2
  spline S219 degree 2 poles (-29.3469, -53.1538) (-29.1838, -53.0747) (-29.0256, -52.7732) (-29.0256, -52.5112) knots 0 0 0 1 2 2 2
  spline S220 degree 2 poles (-29.0256, -52.5112) (-29.0256, -52.2739) (-29.3173, -51.7301) (-29.5941, -51.4434) knots 0 0 0 1 2 2 2
  spline S221 degree 2 poles (-29.5941, -51.4434) (-29.6633, -51.4484) (-29.8561, -51.4583) (-29.9846, -51.4583) knots 0 0 0 1 2 2 2
  line L150 (-29.9846, -51.4583) -> (-33, -51.4583)
  line L151 (-33, -51.4583) -> (-33, -50.6871)
  line L152 (-33, -50.6871) -> (-30.3504, -50.6871)
  spline S222 degree 2 poles (-30.3504, -50.6871) (-30.034, -50.6871) (-29.4952, -50.6377) (-29.3469, -50.5586) knots 0 0 0 1 2 2 2
  spline S223 degree 2 poles (-29.3469, -50.5586) (-29.1838, -50.4795) (-29.0256, -50.178) (-29.0256, -49.916) knots 0 0 0 1 2 2 2
  spline S224 degree 2 poles (-29.0256, -49.916) (-29.0256, -49.6688) (-29.337, -49.1201) (-29.5793, -48.863) knots 0 0 0 1 2 2 2
  line L153 (-29.5793, -48.863) -> (-33, -48.863)
  line L154 (-33, -48.863) -> (-33, -48.0919)
  line L155 (-33, -48.0919) -> (-28.4225, -48.0919)
  line L156 (-28.4225, -48.0919) -> (-28.4225, -48.863)
  line L157 (-28.4225, -48.863) -> (-28.9267, -48.863)
  spline S225 degree 2 poles (-28.9267, -48.863) (-28.6252, -49.1646) (-28.294, -49.7578) (-28.294, -50.1137) knots 0 0 0 1 2 2 2
  spline S226 degree 2 poles (-28.294, -50.1137) (-28.294, -50.519) (-28.6647, -51.1468) (-29.0849, -51.31) knots 0 0 0 1 2 2 2
  spline S227 degree 2 poles (-29.0849, -51.31) (-28.6944, -51.6609) (-28.294, -52.3233) (-28.294, -52.7089) knots 0 0 0 1 2 2 2
  spline S228 degree 2 poles (-28.294, -52.7089) (-28.294, -53.0055) (-28.4769, -53.49) (-28.6845, -53.6679) knots 0 0 0 1 2 2 2
  spline S229 degree 2 poles (-28.6845, -53.6679) (-28.8921, -53.8508) (-29.515, -54.0535) (-29.9846, -54.0535) knots 0 0 0 1 2 2 2
  line L158 (-29.9846, -54.0535) -> (-33, -54.0535)
  line L159 (-33, -54.0535) -> (-33, -53.2823)
  line L160 (-33, -60.3265) -> (-30.3504, -60.3265)
  spline S230 degree 2 poles (-30.3504, -60.3265) (-30.034, -60.3265) (-29.4952, -60.2771) (-29.3469, -60.198) knots 0 0 0 1 2 2 2
  spline S231 degree 2 poles (-29.3469, -60.198) (-29.1838, -60.1189) (-29.0256, -59.8173) (-29.0256, -59.5553) knots 0 0 0 1 2 2 2
  spline S232 degree 2 poles (-29.0256, -59.5553) (-29.0256, -59.3181) (-29.3173, -58.7743) (-29.5941, -58.4876) knots 0 0 0 1 2 2 2
  spline S233 degree 2 poles (-29.5941, -58.4876) (-29.6633, -58.4925) (-29.8561, -58.5024) (-29.9846, -58.5024) knots 0 0 0 1 2 2 2
  line L161 (-29.9846, -58.5024) -> (-33, -58.5024)
  line L162 (-33, -58.5024) -> (-33, -57.7313)
  line L163 (-33, -57.7313) -> (-30.3504, -57.7313)
  spline S234 degree 2 poles (-30.3504, -57.7313) (-30.034, -57.7313) (-29.4952, -57.6818) (-29.3469, -57.6028) knots 0 0 0 1 2 2 2
  spline S235 degree 2 poles (-29.3469, -57.6028) (-29.1838, -57.5237) (-29.0256, -57.2221) (-29.0256, -56.9601) knots 0 0 0 1 2 2 2
  spline S236 degree 2 poles (-29.0256, -56.9601) (-29.0256, -56.713) (-29.337, -56.1643) (-29.5793, -55.9072) knots 0 0 0 1 2 2 2
  line L164 (-29.5793, -55.9072) -> (-33, -55.9072)
  line L165 (-33, -55.9072) -> (-33, -55.1361)
  line L166 (-33, -55.1361) -> (-28.4225, -55.1361)
  line L167 (-28.4225, -55.1361) -> (-28.4225, -55.9072)
  line L168 (-28.4225, -55.9072) -> (-28.9267, -55.9072)
  spline S237 degree 2 poles (-28.9267, -55.9072) (-28.6252, -56.2088) (-28.294, -56.8019) (-28.294, -57.1579) knots 0 0 0 1 2 2 2
  spline S238 degree 2 poles (-28.294, -57.1579) (-28.294, -57.5632) (-28.6647, -58.191) (-29.0849, -58.3541) knots 0 0 0 1 2 2 2
  spline S239 degree 2 poles (-29.0849, -58.3541) (-28.6944, -58.7051) (-28.294, -59.3675) (-28.294, -59.7531) knots 0 0 0 1 2 2 2
  spline S240 degree 2 poles (-28.294, -59.7531) (-28.294, -60.0497) (-28.4769, -60.5341) (-28.6845, -60.7121) knots 0 0 0 1 2 2 2
  spline S241 degree 2 poles (-28.6845, -60.7121) (-28.8921, -60.895) (-29.515, -61.0976) (-29.9846, -61.0976) knots 0 0 0 1 2 2 2
  line L169 (-29.9846, -61.0976) -> (-33, -61.0976)
  line L170 (-33, -61.0976) -> (-33, -60.3265)
  line L171 (-37.8145, -42.6543) -> (-43, -40.0146)
  line L172 (-43, -40.0146) -> (-43, -39.1446)
  line L173 (-43, -39.1446) -> (-37.6168, -41.9326)
  line L174 (-37.6168, -41.9326) -> (-37.6168, -38.7837)
  line L175 (-37.6168, -38.7837) -> (-36.9, -38.7837)
  line L176 (-36.9, -38.7837) -> (-36.9, -42.6543)
  line L177 (-36.9, -42.6543) -> (-37.8145, -42.6543)
  spline S242 degree 2 poles (-39.95, -47.1972) (-41.5912, -47.1972) (-43.1285, -46.2431) (-43.1285, -45.2495) knots 0 0 0 1 2 2 2
  spline S243 degree 2 poles (-43.1285, -45.2495) (-43.1285, -44.2411) (-41.5615, -43.2969) (-39.9549, -43.2969) knots 0 0 0 1 2 2 2
  spline S244 degree 2 poles (-39.9549, -43.2969) (-38.3039, -43.2969) (-36.7764, -44.251) (-36.7764, -45.2495) knots 0 0 0 1 2 2 2
  spline S245 degree 2 poles (-36.7764, -45.2495) (-36.7764, -46.253) (-38.3583, -47.1972) (-39.95, -47.1972) knots 0 0 0 1 2 2 2
  spline S246 degree 2 poles (-41.8087, -46.1492) (-41.5071, -46.2678) (-40.5778, -46.3667) (-39.95, -46.3667) knots 0 0 0 1 2 2 2
  spline S247 degree 2 poles (-39.95, -46.3667) (-39.3222, -46.3667) (-38.3978, -46.2678) (-38.0864, -46.1442) knots 0 0 0 1 2 2 2
  spline S248 degree 2 poles (-38.0864, -46.1442) (-37.775, -46.0207) (-37.4536, -45.5906) (-37.4536, -45.2495) knots 0 0 0 1 2 2 2
  spline S249 degree 2 poles (-37.4536, -45.2495) (-37.4536, -44.9084) (-37.775, -44.4685) (-38.0963, -44.34) knots 0 0 0 1 2 2 2
  spline S250 degree 2 poles (-38.0963, -44.34) (-38.4077, -44.2164) (-39.3568, -44.1274) (-39.9549, -44.1274) knots 0 0 0 1 2 2 2
  spline S251 degree 2 poles (-39.9549, -44.1274) (-40.5976, -44.1274) (-41.4577, -44.2065) (-41.7938, -44.335) knots 0 0 0 1 2 2 2
  spline S252 degree 2 poles (-41.7938, -44.335) (-42.1102, -44.4536) (-42.4513, -44.8936) (-42.4513, -45.2495) knots 0 0 0 1 2 2 2
  spline S253 degree 2 poles (-42.4513, -45.2495) (-42.4513, -45.5857) (-42.13, -46.0256) (-41.8087, -46.1492) knots 0 0 0 1 2 2 2
  line L178 (-43, -53.2823) -> (-40.3504, -53.2823)
  spline S254 degree 2 poles (-40.3504, -53.2823) (-40.034, -53.2823) (-39.4952, -53.2329) (-39.3469, -53.1538) knots 0 0 0 1 2 2 2
  spline S255 degree 2 poles (-39.3469, -53.1538) (-39.1838, -53.0747) (-39.0256, -52.7732) (-39.0256, -52.5112) knots 0 0 0 1 2 2 2
  spline S256 degree 2 poles (-39.0256, -52.5112) (-39.0256, -52.2739) (-39.3173, -51.7301) (-39.5941, -51.4434) knots 0 0 0 1 2 2 2
  spline S257 degree 2 poles (-39.5941, -51.4434) (-39.6633, -51.4484) (-39.8561, -51.4583) (-39.9846, -51.4583) knots 0 0 0 1 2 2 2
  line L179 (-39.9846, -51.4583) -> (-43, -51.4583)
  line L180 (-43, -51.4583) -> (-43, -50.6871)
  line L181 (-43, -50.6871) -> (-40.3504, -50.6871)
  spline S258 degree 2 poles (-40.3504, -50.6871) (-40.034, -50.6871) (-39.4952, -50.6377) (-39.3469, -50.5586) knots 0 0 0 1 2 2 2
  spline S259 degree 2 poles (-39.3469, -50.5586) (-39.1838, -50.4795) (-39.0256, -50.178) (-39.0256, -49.916) knots 0 0 0 1 2 2 2
  spline S260 degree 2 poles (-39.0256, -49.916) (-39.0256, -49.6688) (-39.337, -49.1201) (-39.5793, -48.863) knots 0 0 0 1 2 2 2
  line L182 (-39.5793, -48.863) -> (-43, -48.863)
  line L183 (-43, -48.863) -> (-43, -48.0919)
  line L184 (-43, -48.0919) -> (-38.4225, -48.0919)
  line L185 (-38.4225, -48.0919) -> (-38.4225, -48.863)
  line L186 (-38.4225, -48.863) -> (-38.9267, -48.863)
  spline S261 degree 2 poles (-38.9267, -48.863) (-38.6252, -49.1646) (-38.294, -49.7578) (-38.294, -50.1137) knots 0 0 0 1 2 2 2
  spline S262 degree 2 poles (-38.294, -50.1137) (-38.294, -50.519) (-38.6647, -51.1468) (-39.0849, -51.31) knots 0 0 0 1 2 2 2
  spline S263 degree 2 poles (-39.0849, -51.31) (-38.6944, -51.6609) (-38.294, -52.3233) (-38.294, -52.7089) knots 0 0 0 1 2 2 2
  spline S264 degree 2 poles (-38.294, -52.7089) (-38.294, -53.0055) (-38.4769, -53.49) (-38.6845, -53.6679) knots 0 0 0 1 2 2 2
  spline S265 degree 2 poles (-38.6845, -53.6679) (-38.8921, -53.8508) (-39.515, -54.0535) (-39.9846, -54.0535) knots 0 0 0 1 2 2 2
  line L187 (-39.9846, -54.0535) -> (-43, -54.0535)
  line L188 (-43, -54.0535) -> (-43, -53.2823)
  line L189 (-43, -60.3265) -> (-40.3504, -60.3265)